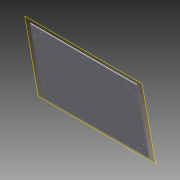
# Autodesk Inventor part: Panel_bottom
Saved by Autodesk Inventor 2013 (Build 170138000, 138)
## iProperties
Created: 2013-02-02
Part Number: Panel_bottom
Material: Aluminum 6061
Document SubType Name: Modeling
Designer: xylzlyx
Density: 1 g/cm^3
Author: xylzlyx
Autodesk Inventor part; units mm, degrees
ref_plane "YZ Plane" through (0, 0, 0) normal (1, 0, 0) x (0, 1, 0)
ref_plane "XZ Plane" through (0, 0, 0) normal (0, 1, 0) x (-1, 0, 0)
ref_plane "XY Plane" through (0, 0, 0) normal (0, 0, 1) x (1, 0, 0)
ref_plane "10DegOffset" through (-190.5, -127, 0) normal (0, -0.1736482, 0.9848078) x (1, 0, 0)
sketch "BottomDimensions" plane through (-190.5, -127, 0) normal (0, -0.1736482, 0.9848078) x (1, 0, 0)
  line L0 (380, 250.1412) -> (1, 250.1412) construction
  line L1 (0, 249.1564) -> (0, 0.9848) construction
  line L2 (381, 0.9848) -> (381, 249.1564) construction
  line L3 (1, 0) -> (380, 0) construction
  line L4 (0, 250.1412) -> (381, 250.1412)
  line L5 (381, 250.1412) -> (381, 0)
  line L6 (381, 0) -> (0, 0)
  line L7 (0, 0) -> (0, 250.1412)
  point P0 (190.5, 125.0706)
  constraints: 8 end point, 2 horizontal alignment, 2 parallel, 2 vertical alignment, 1 horizontal, 1 perpendicular
extrude "Extrusion1" add sketch "BottomDimensions" along normal blind 3.175
fillet "Fillet1" radius 1 4 edges at (-190.5, 119.0653, 44.9999) (190.5, 119.0653, 44.9999) (190.5, -127.2757, 1.5634) (-190.5, -127.2757, 1.5634)
sketch "ScrewHoleSketch" plane through (-190.5, -127.5513, 3.1268) normal (0, -0.1736482, 0.9848078) x (1, 0, 0)
  line L0 (9.525, 40.9987) -> (12.7, 40.9987) projected
  line L1 (12.7, 37.2014) -> (9.525, 37.2014) projected
  line L2 (12.7, 209.1425) -> (9.525, 209.1425) projected
  line L3 (9.525, 212.9398) -> (12.7, 212.9398) projected
  line L4 (39.9986, 240.6162) -> (39.9986, 237.4412) projected
  line L5 (36.2013, 237.4412) -> (36.2013, 240.6162) projected
  line L6 (188.6014, 237.4412) -> (188.6014, 240.6162) projected
  line L7 (192.3987, 240.6162) -> (192.3987, 237.4412) projected
  line L8 (344.7986, 240.6162) -> (344.7986, 237.4412) projected
  line L9 (341.0013, 237.4412) -> (341.0013, 240.6162) projected
  line L10 (371.475, 209.1425) -> (368.3, 209.1425) projected
  line L11 (368.3, 212.9398) -> (371.475, 212.9398) projected
  line L12 (368.3, 40.9986) -> (371.475, 40.9986) projected
  line L13 (371.475, 37.2013) -> (368.3, 37.2013) projected
  line L14 (341.0014, 9.525) -> (341.0014, 12.7) projected
  line L15 (344.7987, 12.7) -> (344.7987, 9.525) projected
  line L16 (192.3987, 12.7) -> (192.3987, 9.525) projected
  line L17 (188.6014, 9.525) -> (188.6014, 12.7) projected
  line L18 (36.2013, 9.525) -> (36.2013, 12.7) projected
  line L19 (39.9986, 12.7) -> (39.9986, 9.525) projected
  line L20 (9.525, 212.9398) -> (9.525, 209.1425) construction
  line L21 (39.9986, 240.6162) -> (36.2013, 240.6162) construction
  line L22 (192.3987, 240.6162) -> (188.6014, 240.6162) construction
  line L23 (344.7986, 240.6162) -> (341.0013, 240.6162) construction
  line L24 (371.475, 209.1425) -> (371.475, 212.9398) construction
  line L25 (368.3, 40.9986) -> (368.3, 37.2013) construction
  line L26 (344.7987, 12.7) -> (341.0014, 12.7) construction
  line L27 (192.3987, 12.7) -> (188.6014, 12.7) construction
  line L28 (36.2013, 9.525) -> (39.9986, 9.525) construction
  line L29 (12.7, 37.2014) -> (12.7, 40.9987) construction
  point P0 (190.5, 125.0706)
  point P1 (11.1125, 211.0412)
  point P2 (38.1, 239.0287)
  point P3 (190.5, 239.0287)
  point P4 (342.9, 239.0287)
  point P5 (369.8875, 211.0412)
  point P6 (369.8875, 39.1)
  point P7 (342.9, 11.1125)
  point P8 (36.2013, 239.0287)
  point P9 (9.525, 211.0412)
  point P10 (38.1, 240.6162)
  point P11 (11.1125, 212.9398)
  point P12 (190.5, 240.6162)
  point P13 (192.3987, 239.0287)
  point P14 (344.7986, 239.0287)
  point P15 (342.9, 240.6162)
  point P16 (369.8875, 212.9398)
  point P17 (371.475, 211.0412)
  point P18 (368.3, 39.1)
  point P19 (341.0014, 11.1125)
  point P20 (369.8875, 40.9986)
  point P21 (342.9, 12.7)
  point P22 (11.1125, 39.1)
  point P23 (38.1, 11.1125)
  point P24 (190.5, 11.1125)
  point P25 (188.6014, 11.1125)
  point P26 (190.5, 12.7)
  point P27 (38.1, 9.525)
  point P28 (11.1125, 37.2014)
  point P29 (12.7, 39.1)
  point P30 (36.2013, 11.1125)
  constraints: 20 end point, 20 midpoint, 10 horizontal alignment, 10 vertical alignment, 3 parallel
hole "Hole1" at (-179.3875, 80.2836, 39.7737) at (-152.4, 107.846, 44.6337) at (0, 107.846, 44.6337) at (152.4, 107.846, 44.6337) at (179.3875, 80.2836, 39.7737) at (179.3875, -89.0453, 9.9164) at (152.4, -116.6077, 5.0564) at (-179.3875, -89.0453, 9.9164) at (-152.4, -116.6077, 5.0564) at (0, -116.6077, 5.0564) direction (0, 0.1736482, -0.9848078) diameter 3.7973 end through all
equation "\"d3\" = ScrewHoleD"
equation "\"ScrewHoleD\" = 3.7973"
body "Solid1"
